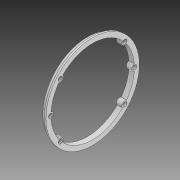
# Autodesk Inventor part: SwivelMountClamp
Saved by Autodesk Inventor 2020 (Build 240168000, 168)
## iProperties
Created: 2020-09-19
Part Number: SwivelMountClamp
Material: Generic
Document SubType Name: Modeling
Designer: DDeGo
Density: 1 g/cm^3
Appearance: Default
Author: DDeGo
Autodesk Inventor part; units mm, degrees
ref_plane "YZ Plane" through (0, 0, 0) normal (1, 0, 0) x (0, 1, 0)
ref_plane "XZ Plane" through (0, 0, 0) normal (0, 1, 0) x (-1, 0, 0)
ref_plane "XY Plane" through (0, 0, 0) normal (0, 0, 1) x (1, 0, 0)
sketch "Sketch1" plane through (0, 0, 0) normal (0, 0, 1) x (1, 0, 0)
  line L0 (0, 0) -> (0, -59.4) construction
  line L1 (0, -59.4) -> (7.5, -59.4)
  line L2 (7.5, -59.4) -> (7.5, -66.4)
  line L3 (7.5, -66.4) -> (5, -66.4)
  line L4 (5, -66.4) -> (5, -63.4)
  line L5 (5, -63.4) -> (0, -63.4)
  line L6 (0, -63.4) -> (0, -59.4)
  line L7 (0, 0) -> (7.5, 0) construction
  line L8 (7.5, 0) -> (7.5, -59.4) construction
  line L9 (7.5, -59.4) -> (7.5, -66.4)
  dimension "d0" = 63.4
  dimension "d1" = 4
  dimension "d2" = 2.5
  dimension "d3" = 3
  dimension "d4" = 5
  constraints: 20 end point, 7 perpendicular, 1 coincident, 1 collinear, 1 horizontal, 1 point on line, 1 vertical
  measures "d0" distance from line of L7.start L5
  measures "d1" distance between parallel lines of L1 L5
  measures "d2" distance between parallel lines of L2 L4
  measures "d3" distance of L3.end L4.end
  measures "d4" distance of L4.end L5.end
revolve "Revolution1" add sketch "Sketch1" angle 360 about axis through (0, 0, 0) along (1, 0, 0)
sketch "Sketch2" plane through (0, 0, 0) normal (-1, 0, 0) x (0, 0, 1)
  line L0 (0, 0) -> (0, 55.6716) construction
  line L1 (0, 0) -> (-59.868, 0) construction
  line L2 (0, 0) -> (-47.9174, -40.2075) construction
  line L3 (0, 0) -> (-42.8366, 35.9442) construction
  circle A0 centre (-45.8861, 38.503) radius 3.5 construction
  circle A1 centre (-59.9, 0) radius 3.5 construction
  circle A2 centre (-45.8861, -38.503) radius 3.5 construction
  circle A3 centre (-45.8861, 38.503) radius 1.75
  circle A4 centre (-45.8861, 38.503) radius 4.5
  circle A5 centre (-59.9, 0) radius 4.5
  circle A6 centre (-59.9, 0) radius 1.75
  circle A7 centre (-45.8861, -38.503) radius 1.75
  circle A8 centre (-45.8861, -38.503) radius 4.5
  circle A9 centre (0, 0) radius 63.4 projected
  circle A10 centre (45.8861, 38.503) radius 1.75
  circle A11 centre (45.8861, 38.503) radius 3.5 construction
  circle A12 centre (45.8861, 38.503) radius 4.5
  circle A13 centre (59.9, 0) radius 1.75
  circle A14 centre (59.9, 0) radius 4.5
  circle A15 centre (59.9, 0) radius 3.5 construction
  circle A16 centre (45.8861, -38.503) radius 3.5 construction
  circle A17 centre (45.8861, -38.503) radius 1.75
  circle A18 centre (45.8861, -38.503) radius 4.5
  point P0 (-24.75, 53.9981)
  point P1 (-57.3891, -15.325)
  point P2 (57.3891, -15.325)
  point P3 (42.8366, 35.9442)
  point P4 (59.868, 0)
  point P5 (47.9174, -40.2075)
  point P6 (-46.6461, 42.9383)
  point P7 (-50.386, 38.4813)
  point P8 (-63.3332, 2.9091)
  point P9 (-63.3332, -2.9091)
  point P10 (-50.386, -38.4813)
  point P11 (-46.6461, -42.9383)
  point P12 (46.6461, 42.9383)
  point P13 (50.386, 38.4813)
  point P14 (63.3332, 2.9091)
  point P15 (63.3332, -2.9091)
  point P16 (50.386, -38.4813)
  point P17 (46.6461, -42.9383)
  dimension "d9" = 40
  dimension "d10" = 40
  dimension "d11" = 7
  dimension "d12" = 9
  dimension "d13" = 3.5
  constraints: 18 centre point, 14 coincident, 13 symmetric about line, 8 end point, 6 equal radius, 3 point on line, 3 tangent, 1 horizontal, 1 vertical, 9 other
  measures "d9" angle of L3 L1
  measures "d10" angle of L2 L1
  measures "d11" diameter of A0
  measures "d12" diameter of A8
  measures "d13" diameter of A7
extrude "Extrusion1" add sketch "Sketch2" against normal up to surface (7.5 mm away) contours A4 A9 | A9 A12 | A5 A9 | A9 A14 | A8 A9 | A9 A18 picked at (-46.8937, 41.5565) picked at (46.8937, 41.5565) picked at (-62.6452, -1.6799) picked at (62.3698, 2.2508) picked at (-46.8937, -41.5565) picked at (46.8937, -41.5565)
extrude "Extrusion2" cut sketch "Sketch2" against normal through all contours A3 | A6 | A7 | A10 | A13 | A17
sketch "Sketch3" plane through (7.5, 0, 0) normal (1, 0, 0) x (0, 0, -1)
  circle A0 centre (-45.8861, 38.503) radius 1.75 projected
  circle A1 centre (-45.8861, 38.503) radius 3
  circle A2 centre (-59.9, 0) radius 1.75 projected
  circle A3 centre (-59.9, 0) radius 3
  circle A4 centre (-45.8861, -38.503) radius 1.75 projected
  circle A5 centre (-45.8861, -38.503) radius 3
  circle A6 centre (45.8861, -38.503) radius 1.75 projected
  circle A7 centre (45.8861, -38.503) radius 3
  circle A8 centre (59.9, 0) radius 1.75 projected
  circle A9 centre (59.9, 0) radius 3
  circle A10 centre (45.8861, 38.503) radius 1.75 projected
  circle A11 centre (45.8861, 38.503) radius 3
  point P0 (0, 0)
  dimension "d18" = 6
  constraints: 6 centre point, 6 coincident, 5 equal radius
  measures "d18" diameter of A1
extrude "Extrusion3" cut sketch "Sketch3" against normal blind 3 contours A0 | A1 | A2 | A3 | A4 | A5 | A6 | A7 | A8 | A9 | A10 | A11
equation "\"d10\" = d9"
body "Solid1"
